Autodesk Inventor part; units mm, degrees
(part 3 of 4)
sketch "Sketch3" plane through (0, 0, 15) normal (0, 0, 1) x (1, 0, 0)
  line L0 (0, 0) -> (0, 2.4)
  line L1 (0, 2.4) -> (-384, 2.4)
  line L2 (-384, 2.4) -> (-384, 0)
  arc A0 (-384, 0) -> (-383.1122, 0.9525) centre (-384, 0.89) ccw
  arc A1 (-382.8628, 1.22) -> (-383.1122, 0.9525) centre (-382.8628, 0.97) ccw
  line L3 (-382.8628, 1.22) -> (-382.1372, 1.22)
  arc A2 (-381.8878, 0.9525) -> (-382.1372, 1.22) centre (-382.1372, 0.97) ccw
  arc A3 (-381.8878, 0.9525) -> (-380.1122, 0.9525) centre (-381, 0.89) ccw
  arc A4 (-379.8628, 1.22) -> (-380.1122, 0.9525) centre (-379.8628, 0.97) ccw
  line L4 (-379.8628, 1.22) -> (-379.1372, 1.22)
  arc A5 (-378.8878, 0.9525) -> (-379.1372, 1.22) centre (-379.1372, 0.97) ccw
  arc A6 (-378.8878, 0.9525) -> (-377.1122, 0.9525) centre (-378, 0.89) ccw
  arc A7 (-376.8628, 1.22) -> (-377.1122, 0.9525) centre (-376.8628, 0.97) ccw
  line L5 (-376.8628, 1.22) -> (-376.1372, 1.22)
  arc A8 (-375.8878, 0.9525) -> (-376.1372, 1.22) centre (-376.1372, 0.97) ccw
  arc A9 (-375.8878, 0.9525) -> (-374.1122, 0.9525) centre (-375, 0.89) ccw
  arc A10 (-373.8628, 1.22) -> (-374.1122, 0.9525) centre (-373.8628, 0.97) ccw
  line L6 (-373.8628, 1.22) -> (-373.1372, 1.22)
  arc A11 (-372.8878, 0.9525) -> (-373.1372, 1.22) centre (-373.1372, 0.97) ccw
  arc A12 (-372.8878, 0.9525) -> (-371.1122, 0.9525) centre (-372, 0.89) ccw
  arc A13 (-370.8628, 1.22) -> (-371.1122, 0.9525) centre (-370.8628, 0.97) ccw
  line L7 (-370.8628, 1.22) -> (-370.1372, 1.22)
  arc A14 (-369.8878, 0.9525) -> (-370.1372, 1.22) centre (-370.1372, 0.97) ccw
  arc A15 (-369.8878, 0.9525) -> (-368.1122, 0.9525) centre (-369, 0.89) ccw
  arc A16 (-367.8628, 1.22) -> (-368.1122, 0.9525) centre (-367.8628, 0.97) ccw
  line L8 (-367.8628, 1.22) -> (-367.1372, 1.22)
  arc A17 (-366.8878, 0.9525) -> (-367.1372, 1.22) centre (-367.1372, 0.97) ccw
  arc A18 (-366.8878, 0.9525) -> (-365.1122, 0.9525) centre (-366, 0.89) ccw
  arc A19 (-364.8628, 1.22) -> (-365.1122, 0.9525) centre (-364.8628, 0.97) ccw
  line L9 (-364.8628, 1.22) -> (-364.1372, 1.22)
  arc A20 (-363.8878, 0.9525) -> (-364.1372, 1.22) centre (-364.1372, 0.97) ccw
  arc A21 (-363.8878, 0.9525) -> (-362.1122, 0.9525) centre (-363, 0.89) ccw
  arc A22 (-361.8628, 1.22) -> (-362.1122, 0.9525) centre (-361.8628, 0.97) ccw
  line L10 (-361.8628, 1.22) -> (-361.1372, 1.22)
  arc A23 (-360.8878, 0.9525) -> (-361.1372, 1.22) centre (-361.1372, 0.97) ccw
  arc A24 (-360.8878, 0.9525) -> (-359.1122, 0.9525) centre (-360, 0.89) ccw
  arc A25 (-358.8628, 1.22) -> (-359.1122, 0.9525) centre (-358.8628, 0.97) ccw
  line L11 (-358.8628, 1.22) -> (-358.1372, 1.22)
  arc A26 (-357.8878, 0.9525) -> (-358.1372, 1.22) centre (-358.1372, 0.97) ccw
  arc A27 (-357.8878, 0.9525) -> (-356.1122, 0.9525) centre (-357, 0.89) ccw
  arc A28 (-355.8628, 1.22) -> (-356.1122, 0.9525) centre (-355.8628, 0.97) ccw
  line L12 (-355.8628, 1.22) -> (-355.1372, 1.22)
  arc A29 (-354.8878, 0.9525) -> (-355.1372, 1.22) centre (-355.1372, 0.97) ccw
  arc A30 (-354.8878, 0.9525) -> (-353.1122, 0.9525) centre (-354, 0.89) ccw
  arc A31 (-352.8628, 1.22) -> (-353.1122, 0.9525) centre (-352.8628, 0.97) ccw
  line L13 (-352.8628, 1.22) -> (-352.1372, 1.22)
  arc A32 (-351.8878, 0.9525) -> (-352.1372, 1.22) centre (-352.1372, 0.97) ccw
  arc A33 (-351.8878, 0.9525) -> (-350.1122, 0.9525) centre (-351, 0.89) ccw
  arc A34 (-349.8628, 1.22) -> (-350.1122, 0.9525) centre (-349.8628, 0.97) ccw
  line L14 (-349.8628, 1.22) -> (-349.1372, 1.22)
  arc A35 (-348.8878, 0.9525) -> (-349.1372, 1.22) centre (-349.1372, 0.97) ccw
  arc A36 (-348.8878, 0.9525) -> (-347.1122, 0.9525) centre (-348, 0.89) ccw
  arc A37 (-346.8628, 1.22) -> (-347.1122, 0.9525) centre (-346.8628, 0.97) ccw
  line L15 (-346.8628, 1.22) -> (-346.1372, 1.22)
  arc A38 (-345.8878, 0.9525) -> (-346.1372, 1.22) centre (-346.1372, 0.97) ccw
  arc A39 (-345.8878, 0.9525) -> (-344.1122, 0.9525) centre (-345, 0.89) ccw
  arc A40 (-343.8628, 1.22) -> (-344.1122, 0.9525) centre (-343.8628, 0.97) ccw
  line L16 (-343.8628, 1.22) -> (-343.1372, 1.22)
  arc A41 (-342.8878, 0.9525) -> (-343.1372, 1.22) centre (-343.1372, 0.97) ccw
  arc A42 (-342.8878, 0.9525) -> (-341.1122, 0.9525) centre (-342, 0.89) ccw
  arc A43 (-340.8628, 1.22) -> (-341.1122, 0.9525) centre (-340.8628, 0.97) ccw
  line L17 (-340.8628, 1.22) -> (-340.1372, 1.22)
  arc A44 (-339.8878, 0.9525) -> (-340.1372, 1.22) centre (-340.1372, 0.97) ccw
  arc A45 (-339.8878, 0.9525) -> (-338.1122, 0.9525) centre (-339, 0.89) ccw
  arc A46 (-337.8628, 1.22) -> (-338.1122, 0.9525) centre (-337.8628, 0.97) ccw
  line L18 (-337.8628, 1.22) -> (-337.1372, 1.22)
  arc A47 (-336.8878, 0.9525) -> (-337.1372, 1.22) centre (-337.1372, 0.97) ccw
  arc A48 (-336.8878, 0.9525) -> (-335.1122, 0.9525) centre (-336, 0.89) ccw
  arc A49 (-334.8628, 1.22) -> (-335.1122, 0.9525) centre (-334.8628, 0.97) ccw
  line L19 (-334.8628, 1.22) -> (-334.1372, 1.22)
  arc A50 (-333.8878, 0.9525) -> (-334.1372, 1.22) centre (-334.1372, 0.97) ccw
  arc A51 (-333.8878, 0.9525) -> (-332.1122, 0.9525) centre (-333, 0.89) ccw
  arc A52 (-331.8628, 1.22) -> (-332.1122, 0.9525) centre (-331.8628, 0.97) ccw
  line L20 (-331.8628, 1.22) -> (-331.1372, 1.22)
  arc A53 (-330.8878, 0.9525) -> (-331.1372, 1.22) centre (-331.1372, 0.97) ccw
  arc A54 (-330.8878, 0.9525) -> (-329.1122, 0.9525) centre (-330, 0.89) ccw
  arc A55 (-328.8628, 1.22) -> (-329.1122, 0.9525) centre (-328.8628, 0.97) ccw
  line L21 (-328.8628, 1.22) -> (-328.1372, 1.22)
  arc A56 (-327.8878, 0.9525) -> (-328.1372, 1.22) centre (-328.1372, 0.97) ccw
  arc A57 (-327.8878, 0.9525) -> (-326.1122, 0.9525) centre (-327, 0.89) ccw
  arc A58 (-325.8628, 1.22) -> (-326.1122, 0.9525) centre (-325.8628, 0.97) ccw
  line L22 (-325.8628, 1.22) -> (-325.1372, 1.22)
  arc A59 (-324.8878, 0.9525) -> (-325.1372, 1.22) centre (-325.1372, 0.97) ccw
  arc A60 (-324.8878, 0.9525) -> (-323.1122, 0.9525) centre (-324, 0.89) ccw
  arc A61 (-322.8628, 1.22) -> (-323.1122, 0.9525) centre (-322.8628, 0.97) ccw
  line L23 (-322.8628, 1.22) -> (-322.1372, 1.22)
  arc A62 (-321.8878, 0.9525) -> (-322.1372, 1.22) centre (-322.1372, 0.97) ccw
  arc A63 (-321.8878, 0.9525) -> (-320.1122, 0.9525) centre (-321, 0.89) ccw
  arc A64 (-319.8628, 1.22) -> (-320.1122, 0.9525) centre (-319.8628, 0.97) ccw
  line L24 (-319.8628, 1.22) -> (-319.1372, 1.22)
  arc A65 (-318.8878, 0.9525) -> (-319.1372, 1.22) centre (-319.1372, 0.97) ccw
  arc A66 (-318.8878, 0.9525) -> (-317.1122, 0.9525) centre (-318, 0.89) ccw
  arc A67 (-316.8628, 1.22) -> (-317.1122, 0.9525) centre (-316.8628, 0.97) ccw
  line L25 (-316.8628, 1.22) -> (-316.1372, 1.22)
  arc A68 (-315.8878, 0.9525) -> (-316.1372, 1.22) centre (-316.1372, 0.97) ccw
  arc A69 (-315.8878, 0.9525) -> (-314.1122, 0.9525) centre (-315, 0.89) ccw
  arc A70 (-313.8628, 1.22) -> (-314.1122, 0.9525) centre (-313.8628, 0.97) ccw
  line L26 (-313.8628, 1.22) -> (-313.1372, 1.22)
  arc A71 (-312.8878, 0.9525) -> (-313.1372, 1.22) centre (-313.1372, 0.97) ccw
  arc A72 (-312.8878, 0.9525) -> (-311.1122, 0.9525) centre (-312, 0.89) ccw
  arc A73 (-310.8628, 1.22) -> (-311.1122, 0.9525) centre (-310.8628, 0.97) ccw
  line L27 (-310.8628, 1.22) -> (-310.1372, 1.22)
  arc A74 (-309.8878, 0.9525) -> (-310.1372, 1.22) centre (-310.1372, 0.97) ccw
  arc A75 (-309.8878, 0.9525) -> (-308.1122, 0.9525) centre (-309, 0.89) ccw
  arc A76 (-307.8628, 1.22) -> (-308.1122, 0.9525) centre (-307.8628, 0.97) ccw
  line L28 (-307.8628, 1.22) -> (-307.1372, 1.22)
  arc A77 (-306.8878, 0.9525) -> (-307.1372, 1.22) centre (-307.1372, 0.97) ccw
  arc A78 (-306.8878, 0.9525) -> (-305.1122, 0.9525) centre (-306, 0.89) ccw
  arc A79 (-304.8628, 1.22) -> (-305.1122, 0.9525) centre (-304.8628, 0.97) ccw
  line L29 (-304.8628, 1.22) -> (-304.1372, 1.22)
  arc A80 (-303.8878, 0.9525) -> (-304.1372, 1.22) centre (-304.1372, 0.97) ccw
  arc A81 (-303.8878, 0.9525) -> (-302.1122, 0.9525) centre (-303, 0.89) ccw
  arc A82 (-301.8628, 1.22) -> (-302.1122, 0.9525) centre (-301.8628, 0.97) ccw
  line L30 (-301.8628, 1.22) -> (-301.1372, 1.22)
  arc A83 (-300.8878, 0.9525) -> (-301.1372, 1.22) centre (-301.1372, 0.97) ccw
  arc A84 (-300.8878, 0.9525) -> (-299.1122, 0.9525) centre (-300, 0.89) ccw
  arc A85 (-298.8628, 1.22) -> (-299.1122, 0.9525) centre (-298.8628, 0.97) ccw
  line L31 (-298.8628, 1.22) -> (-298.1372, 1.22)
  arc A86 (-297.8878, 0.9525) -> (-298.1372, 1.22) centre (-298.1372, 0.97) ccw
  arc A87 (-297.8878, 0.9525) -> (-296.1122, 0.9525) centre (-297, 0.89) ccw
  arc A88 (-295.8628, 1.22) -> (-296.1122, 0.9525) centre (-295.8628, 0.97) ccw
  line L32 (-295.8628, 1.22) -> (-295.1372, 1.22)
  arc A89 (-294.8878, 0.9525) -> (-295.1372, 1.22) centre (-295.1372, 0.97) ccw
  arc A90 (-294.8878, 0.9525) -> (-293.1122, 0.9525) centre (-294, 0.89) ccw
  arc A91 (-292.8628, 1.22) -> (-293.1122, 0.9525) centre (-292.8628, 0.97) ccw
  line L33 (-292.8628, 1.22) -> (-292.1372, 1.22)
  arc A92 (-291.8878, 0.9525) -> (-292.1372, 1.22) centre (-292.1372, 0.97) ccw
  arc A93 (-291.8878, 0.9525) -> (-290.1122, 0.9525) centre (-291, 0.89) ccw
  arc A94 (-289.8628, 1.22) -> (-290.1122, 0.9525) centre (-289.8628, 0.97) ccw
  line L34 (-289.8628, 1.22) -> (-289.1372, 1.22)
  arc A95 (-288.8878, 0.9525) -> (-289.1372, 1.22) centre (-289.1372, 0.97) ccw
  arc A96 (-288.8878, 0.9525) -> (-287.1122, 0.9525) centre (-288, 0.89) ccw
  arc A97 (-286.8628, 1.22) -> (-287.1122, 0.9525) centre (-286.8628, 0.97) ccw
  line L35 (-286.8628, 1.22) -> (-286.1372, 1.22)
  arc A98 (-285.8878, 0.9525) -> (-286.1372, 1.22) centre (-286.1372, 0.97) ccw
  arc A99 (-285.8878, 0.9525) -> (-284.1122, 0.9525) centre (-285, 0.89) ccw
  arc A100 (-283.8628, 1.22) -> (-284.1122, 0.9525) centre (-283.8628, 0.97) ccw
  line L36 (-283.8628, 1.22) -> (-283.1372, 1.22)
  arc A101 (-282.8878, 0.9525) -> (-283.1372, 1.22) centre (-283.1372, 0.97) ccw
  arc A102 (-282.8878, 0.9525) -> (-281.1122, 0.9525) centre (-282, 0.89) ccw
  arc A103 (-280.8628, 1.22) -> (-281.1122, 0.9525) centre (-280.8628, 0.97) ccw
  line L37 (-280.8628, 1.22) -> (-280.1372, 1.22)
  arc A104 (-279.8878, 0.9525) -> (-280.1372, 1.22) centre (-280.1372, 0.97) ccw
  arc A105 (-279.8878, 0.9525) -> (-278.1122, 0.9525) centre (-279, 0.89) ccw
  arc A106 (-277.8628, 1.22) -> (-278.1122, 0.9525) centre (-277.8628, 0.97) ccw
  line L38 (-277.8628, 1.22) -> (-277.1372, 1.22)
  arc A107 (-276.8878, 0.9525) -> (-277.1372, 1.22) centre (-277.1372, 0.97) ccw
  arc A108 (-276.8878, 0.9525) -> (-275.1122, 0.9525) centre (-276, 0.89) ccw
  arc A109 (-274.8628, 1.22) -> (-275.1122, 0.9525) centre (-274.8628, 0.97) ccw
  line L39 (-274.8628, 1.22) -> (-274.1372, 1.22)
  arc A110 (-273.8878, 0.9525) -> (-274.1372, 1.22) centre (-274.1372, 0.97) ccw
  arc A111 (-273.8878, 0.9525) -> (-272.1122, 0.9525) centre (-273, 0.89) ccw
  arc A112 (-271.8628, 1.22) -> (-272.1122, 0.9525) centre (-271.8628, 0.97) ccw
  line L40 (-271.8628, 1.22) -> (-271.1372, 1.22)
  arc A113 (-270.8878, 0.9525) -> (-271.1372, 1.22) centre (-271.1372, 0.97) ccw
  arc A114 (-270.8878, 0.9525) -> (-269.1122, 0.9525) centre (-270, 0.89) ccw
  arc A115 (-268.8628, 1.22) -> (-269.1122, 0.9525) centre (-268.8628, 0.97) ccw
  line L41 (-268.8628, 1.22) -> (-268.1372, 1.22)
  arc A116 (-267.8878, 0.9525) -> (-268.1372, 1.22) centre (-268.1372, 0.97) ccw
  arc A117 (-267.8878, 0.9525) -> (-266.1122, 0.9525) centre (-267, 0.89) ccw
  arc A118 (-265.8628, 1.22) -> (-266.1122, 0.9525) centre (-265.8628, 0.97) ccw
  line L42 (-265.8628, 1.22) -> (-265.1372, 1.22)
  arc A119 (-264.8878, 0.9525) -> (-265.1372, 1.22) centre (-265.1372, 0.97) ccw
  arc A120 (-264.8878, 0.9525) -> (-263.1122, 0.9525) centre (-264, 0.89) ccw
  arc A121 (-262.8628, 1.22) -> (-263.1122, 0.9525) centre (-262.8628, 0.97) ccw
  line L43 (-262.8628, 1.22) -> (-262.1372, 1.22)
  arc A122 (-261.8878, 0.9525) -> (-262.1372, 1.22) centre (-262.1372, 0.97) ccw
  arc A123 (-261.8878, 0.9525) -> (-260.1122, 0.9525) centre (-261, 0.89) ccw
  arc A124 (-259.8628, 1.22) -> (-260.1122, 0.9525) centre (-259.8628, 0.97) ccw
  line L44 (-259.8628, 1.22) -> (-259.1372, 1.22)
  arc A125 (-258.8878, 0.9525) -> (-259.1372, 1.22) centre (-259.1372, 0.97) ccw
  arc A126 (-258.8878, 0.9525) -> (-257.1122, 0.9525) centre (-258, 0.89) ccw
  arc A127 (-256.8628, 1.22) -> (-257.1122, 0.9525) centre (-256.8628, 0.97) ccw
  line L45 (-256.8628, 1.22) -> (-256.1372, 1.22)
  arc A128 (-255.8878, 0.9525) -> (-256.1372, 1.22) centre (-256.1372, 0.97) ccw
  arc A129 (-255.8878, 0.9525) -> (-254.1122, 0.9525) centre (-255, 0.89) ccw
  arc A130 (-253.8628, 1.22) -> (-254.1122, 0.9525) centre (-253.8628, 0.97) ccw
  line L46 (-253.8628, 1.22) -> (-253.1372, 1.22)
  arc A131 (-252.8878, 0.9525) -> (-253.1372, 1.22) centre (-253.1372, 0.97) ccw
  arc A132 (-252.8878, 0.9525) -> (-251.1122, 0.9525) centre (-252, 0.89) ccw
  arc A133 (-250.8628, 1.22) -> (-251.1122, 0.9525) centre (-250.8628, 0.97) ccw
  line L47 (-250.8628, 1.22) -> (-250.1372, 1.22)
  arc A134 (-249.8878, 0.9525) -> (-250.1372, 1.22) centre (-250.1372, 0.97) ccw
  arc A135 (-249.8878, 0.9525) -> (-248.1122, 0.9525) centre (-249, 0.89) ccw
  arc A136 (-247.8628, 1.22) -> (-248.1122, 0.9525) centre (-247.8628, 0.97) ccw
  line L48 (-247.8628, 1.22) -> (-247.1372, 1.22)
  arc A137 (-246.8878, 0.9525) -> (-247.1372, 1.22) centre (-247.1372, 0.97) ccw
  arc A138 (-246.8878, 0.9525) -> (-245.1122, 0.9525) centre (-246, 0.89) ccw
  arc A139 (-244.8628, 1.22) -> (-245.1122, 0.9525) centre (-244.8628, 0.97) ccw
  line L49 (-244.8628, 1.22) -> (-244.1372, 1.22)
  arc A140 (-243.8878, 0.9525) -> (-244.1372, 1.22) centre (-244.1372, 0.97) ccw
  arc A141 (-243.8878, 0.9525) -> (-242.1122, 0.9525) centre (-243, 0.89) ccw
  arc A142 (-241.8628, 1.22) -> (-242.1122, 0.9525) centre (-241.8628, 0.97) ccw
  line L50 (-241.8628, 1.22) -> (-241.1372, 1.22)
  arc A143 (-240.8878, 0.9525) -> (-241.1372, 1.22) centre (-241.1372, 0.97) ccw
  arc A144 (-240.8878, 0.9525) -> (-239.1122, 0.9525) centre (-240, 0.89) ccw
  arc A145 (-238.8628, 1.22) -> (-239.1122, 0.9525) centre (-238.8628, 0.97) ccw
  line L51 (-238.8628, 1.22) -> (-238.1372, 1.22)
  arc A146 (-237.8878, 0.9525) -> (-238.1372, 1.22) centre (-238.1372, 0.97) ccw
  arc A147 (-237.8878, 0.9525) -> (-236.1122, 0.9525) centre (-237, 0.89) ccw
  arc A148 (-235.8628, 1.22) -> (-236.1122, 0.9525) centre (-235.8628, 0.97) ccw
  line L52 (-235.8628, 1.22) -> (-235.1372, 1.22)
  arc A149 (-234.8878, 0.9525) -> (-235.1372, 1.22) centre (-235.1372, 0.97) ccw
  arc A150 (-234.8878, 0.9525) -> (-233.1122, 0.9525) centre (-234, 0.89) ccw
  arc A151 (-232.8628, 1.22) -> (-233.1122, 0.9525) centre (-232.8628, 0.97) ccw
  line L53 (-232.8628, 1.22) -> (-232.1372, 1.22)
  arc A152 (-231.8878, 0.9525) -> (-232.1372, 1.22) centre (-232.1372, 0.97) ccw
  arc A153 (-231.8878, 0.9525) -> (-230.1122, 0.9525) centre (-231, 0.89) ccw
  arc A154 (-229.8628, 1.22) -> (-230.1122, 0.9525) centre (-229.8628, 0.97) ccw
  line L54 (-229.8628, 1.22) -> (-229.1372, 1.22)
  arc A155 (-228.8878, 0.9525) -> (-229.1372, 1.22) centre (-229.1372, 0.97) ccw
  arc A156 (-228.8878, 0.9525) -> (-227.1122, 0.9525) centre (-228, 0.89) ccw
  arc A157 (-226.8628, 1.22) -> (-227.1122, 0.9525) centre (-226.8628, 0.97) ccw
  line L55 (-226.8628, 1.22) -> (-226.1372, 1.22)
  arc A158 (-225.8878, 0.9525) -> (-226.1372, 1.22) centre (-226.1372, 0.97) ccw
  arc A159 (-225.8878, 0.9525) -> (-224.1122, 0.9525) centre (-225, 0.89) ccw
  arc A160 (-223.8628, 1.22) -> (-224.1122, 0.9525) centre (-223.8628, 0.97) ccw
  line L56 (-223.8628, 1.22) -> (-223.1372, 1.22)
  arc A161 (-222.8878, 0.9525) -> (-223.1372, 1.22) centre (-223.1372, 0.97) ccw
  arc A162 (-222.8878, 0.9525) -> (-221.1122, 0.9525) centre (-222, 0.89) ccw
  arc A163 (-220.8628, 1.22) -> (-221.1122, 0.9525) centre (-220.8628, 0.97) ccw
  line L57 (-220.8628, 1.22) -> (-220.1372, 1.22)
  arc A164 (-219.8878, 0.9525) -> (-220.1372, 1.22) centre (-220.1372, 0.97) ccw
  arc A165 (-219.8878, 0.9525) -> (-218.1122, 0.9525) centre (-219, 0.89) ccw
  arc A166 (-217.8628, 1.22) -> (-218.1122, 0.9525) centre (-217.8628, 0.97) ccw
  line L58 (-217.8628, 1.22) -> (-217.1372, 1.22)
  arc A167 (-216.8878, 0.9525) -> (-217.1372, 1.22) centre (-217.1372, 0.97) ccw
  arc A168 (-216.8878, 0.9525) -> (-215.1122, 0.9525) centre (-216, 0.89) ccw
  arc A169 (-214.8628, 1.22) -> (-215.1122, 0.9525) centre (-214.8628, 0.97) ccw
  line L59 (-214.8628, 1.22) -> (-214.1372, 1.22)
  arc A170 (-213.8878, 0.9525) -> (-214.1372, 1.22) centre (-214.1372, 0.97) ccw
  arc A171 (-213.8878, 0.9525) -> (-212.1122, 0.9525) centre (-213, 0.89) ccw
  arc A172 (-211.8628, 1.22) -> (-212.1122, 0.9525) centre (-211.8628, 0.97) ccw
  line L60 (-211.8628, 1.22) -> (-211.1372, 1.22)
  arc A173 (-210.8878, 0.9525) -> (-211.1372, 1.22) centre (-211.1372, 0.97) ccw
  arc A174 (-210.8878, 0.9525) -> (-209.1122, 0.9525) centre (-210, 0.89) ccw
  arc A175 (-208.8628, 1.22) -> (-209.1122, 0.9525) centre (-208.8628, 0.97) ccw
  line L61 (-208.8628, 1.22) -> (-208.1372, 1.22)
  arc A176 (-207.8878, 0.9525) -> (-208.1372, 1.22) centre (-208.1372, 0.97) ccw
  arc A177 (-207.8878, 0.9525) -> (-206.1122, 0.9525) centre (-207, 0.89) ccw
  arc A178 (-205.8628, 1.22) -> (-206.1122, 0.9525) centre (-205.8628, 0.97) ccw
  line L62 (-205.8628, 1.22) -> (-205.1372, 1.22)
  arc A179 (-204.8878, 0.9525) -> (-205.1372, 1.22) centre (-205.1372, 0.97) ccw
  arc A180 (-204.8878, 0.9525) -> (-203.1122, 0.9525) centre (-204, 0.89) ccw
  arc A181 (-202.8628, 1.22) -> (-203.1122, 0.9525) centre (-202.8628, 0.97) ccw
  line L63 (-202.8628, 1.22) -> (-202.1372, 1.22)
  arc A182 (-201.8878, 0.9525) -> (-202.1372, 1.22) centre (-202.1372, 0.97) ccw
  arc A183 (-201.8878, 0.9525) -> (-200.1122, 0.9525) centre (-201, 0.89) ccw
  arc A184 (-199.8628, 1.22) -> (-200.1122, 0.9525) centre (-199.8628, 0.97) ccw
  line L64 (-199.8628, 1.22) -> (-199.1372, 1.22)
  arc A185 (-198.8878, 0.9525) -> (-199.1372, 1.22) centre (-199.1372, 0.97) ccw
  arc A186 (-198.8878, 0.9525) -> (-197.1122, 0.9525) centre (-198, 0.89) ccw
  arc A187 (-196.8628, 1.22) -> (-197.1122, 0.9525) centre (-196.8628, 0.97) ccw
  line L65 (-196.8628, 1.22) -> (-196.1372, 1.22)
  arc A188 (-195.8878, 0.9525) -> (-196.1372, 1.22) centre (-196.1372, 0.97) ccw
  arc A189 (-195.8878, 0.9525) -> (-194.1122, 0.9525) centre (-195, 0.89) ccw
  arc A190 (-193.8628, 1.22) -> (-194.1122, 0.9525) centre (-193.8628, 0.97) ccw
  line L66 (-193.8628, 1.22) -> (-193.1372, 1.22)
  arc A191 (-192.8878, 0.9525) -> (-193.1372, 1.22) centre (-193.1372, 0.97) ccw
  arc A192 (-192.8878, 0.9525) -> (-191.1122, 0.9525) centre (-192, 0.89) ccw
  arc A193 (-190.8628, 1.22) -> (-191.1122, 0.9525) centre (-190.8628, 0.97) ccw
  line L67 (-190.8628, 1.22) -> (-190.1372, 1.22)
  arc A194 (-189.8878, 0.9525) -> (-190.1372, 1.22) centre (-190.1372, 0.97) ccw
  arc A195 (-189.8878, 0.9525) -> (-188.1122, 0.9525) centre (-189, 0.89) ccw
  arc A196 (-187.8628, 1.22) -> (-188.1122, 0.9525) centre (-187.8628, 0.97) ccw
  line L68 (-187.8628, 1.22) -> (-187.1372, 1.22)
  arc A197 (-186.8878, 0.9525) -> (-187.1372, 1.22) centre (-187.1372, 0.97) ccw
  arc A198 (-186.8878, 0.9525) -> (-185.1122, 0.9525) centre (-186, 0.89) ccw
  arc A199 (-184.8628, 1.22) -> (-185.1122, 0.9525) centre (-184.8628, 0.97) ccw
  line L69 (-184.8628, 1.22) -> (-184.1372, 1.22)
  arc A200 (-183.8878, 0.9525) -> (-184.1372, 1.22) centre (-184.1372, 0.97) ccw
  arc A201 (-183.8878, 0.9525) -> (-182.1122, 0.9525) centre (-183, 0.89) ccw
  arc A202 (-181.8628, 1.22) -> (-182.1122, 0.9525) centre (-181.8628, 0.97) ccw
  line L70 (-181.8628, 1.22) -> (-181.1372, 1.22)
  arc A203 (-180.8878, 0.9525) -> (-181.1372, 1.22) centre (-181.1372, 0.97) ccw
  arc A204 (-180.8878, 0.9525) -> (-179.1122, 0.9525) centre (-180, 0.89) ccw
  arc A205 (-178.8628, 1.22) -> (-179.1122, 0.9525) centre (-178.8628, 0.97) ccw
  line L71 (-178.8628, 1.22) -> (-178.1372, 1.22)
  arc A206 (-177.8878, 0.9525) -> (-178.1372, 1.22) centre (-178.1372, 0.97) ccw
  arc A207 (-177.8878, 0.9525) -> (-176.1122, 0.9525) centre (-177, 0.89) ccw
  arc A208 (-175.8628, 1.22) -> (-176.1122, 0.9525) centre (-175.8628, 0.97) ccw
  line L72 (-175.8628, 1.22) -> (-175.1372, 1.22)
  arc A209 (-174.8878, 0.9525) -> (-175.1372, 1.22) centre (-175.1372, 0.97) ccw
  arc A210 (-174.8878, 0.9525) -> (-173.1122, 0.9525) centre (-174, 0.89) ccw
  arc A211 (-172.8628, 1.22) -> (-173.1122, 0.9525) centre (-172.8628, 0.97) ccw
  line L73 (-172.8628, 1.22) -> (-172.1372, 1.22)
  arc A212 (-171.8878, 0.9525) -> (-172.1372, 1.22) centre (-172.1372, 0.97) ccw
  arc A213 (-171.8878, 0.9525) -> (-170.1122, 0.9525) centre (-171, 0.89) ccw
  arc A214 (-169.8628, 1.22) -> (-170.1122, 0.9525) centre (-169.8628, 0.97) ccw
  line L74 (-169.8628, 1.22) -> (-169.1372, 1.22)
  arc A215 (-168.8878, 0.9525) -> (-169.1372, 1.22) centre (-169.1372, 0.97) ccw
  arc A216 (-168.8878, 0.9525) -> (-167.1122, 0.9525) centre (-168, 0.89) ccw
  arc A217 (-166.8628, 1.22) -> (-167.1122, 0.9525) centre (-166.8628, 0.97) ccw
  line L75 (-166.8628, 1.22) -> (-166.1372, 1.22)
  arc A218 (-165.8878, 0.9525) -> (-166.1372, 1.22) centre (-166.1372, 0.97) ccw
  arc A219 (-165.8878, 0.9525) -> (-164.1122, 0.9525) centre (-165, 0.89) ccw
  arc A220 (-163.8628, 1.22) -> (-164.1122, 0.9525) centre (-163.8628, 0.97) ccw
  line L76 (-163.8628, 1.22) -> (-163.1372, 1.22)
  arc A221 (-162.8878, 0.9525) -> (-163.1372, 1.22) centre (-163.1372, 0.97) ccw
  arc A222 (-162.8878, 0.9525) -> (-161.1122, 0.9525) centre (-162, 0.89) ccw
  arc A223 (-160.8628, 1.22) -> (-161.1122, 0.9525) centre (-160.8628, 0.97) ccw
  line L77 (-160.8628, 1.22) -> (-160.1372, 1.22)
  arc A224 (-159.8878, 0.9525) -> (-160.1372, 1.22) centre (-160.1372, 0.97) ccw
  arc A225 (-159.8878, 0.9525) -> (-158.1122, 0.9525) centre (-159, 0.89) ccw
  arc A226 (-157.8628, 1.22) -> (-158.1122, 0.9525) centre (-157.8628, 0.97) ccw
  line L78 (-157.8628, 1.22) -> (-157.1372, 1.22)
  arc A227 (-156.8878, 0.9525) -> (-157.1372, 1.22) centre (-157.1372, 0.97) ccw
  arc A228 (-156.8878, 0.9525) -> (-155.1122, 0.9525) centre (-156, 0.89) ccw
  arc A229 (-154.8628, 1.22) -> (-155.1122, 0.9525) centre (-154.8628, 0.97) ccw
  line L79 (-154.8628, 1.22) -> (-154.1372, 1.22)
  arc A230 (-153.8878, 0.9525) -> (-154.1372, 1.22) centre (-154.1372, 0.97) ccw
  arc A231 (-153.8878, 0.9525) -> (-152.1122, 0.9525) centre (-153, 0.89) ccw
  arc A232 (-151.8628, 1.22) -> (-152.1122, 0.9525) centre (-151.8628, 0.97) ccw
  line L80 (-151.8628, 1.22) -> (-151.1372, 1.22)
  arc A233 (-150.8878, 0.9525) -> (-151.1372, 1.22) centre (-151.1372, 0.97) ccw
  arc A234 (-150.8878, 0.9525) -> (-149.1122, 0.9525) centre (-150, 0.89) ccw
  arc A235 (-148.8628, 1.22) -> (-149.1122, 0.9525) centre (-148.8628, 0.97) ccw
  line L81 (-148.8628, 1.22) -> (-148.1372, 1.22)
  arc A236 (-147.8878, 0.9525) -> (-148.1372, 1.22) centre (-148.1372, 0.97) ccw
  arc A237 (-147.8878, 0.9525) -> (-146.1122, 0.9525) centre (-147, 0.89) ccw
  arc A238 (-145.8628, 1.22) -> (-146.1122, 0.9525) centre (-145.8628, 0.97) ccw
  line L82 (-145.8628, 1.22) -> (-145.1372, 1.22)
  arc A239 (-144.8878, 0.9525) -> (-145.1372, 1.22) centre (-145.1372, 0.97) ccw
  arc A240 (-144.8878, 0.9525) -> (-143.1122, 0.9525) centre (-144, 0.89) ccw
  arc A241 (-142.8628, 1.22) -> (-143.1122, 0.9525) centre (-142.8628, 0.97) ccw
  line L83 (-142.8628, 1.22) -> (-142.1372, 1.22)
  arc A242 (-141.8878, 0.9525) -> (-142.1372, 1.22) centre (-142.1372, 0.97) ccw
  arc A243 (-141.8878, 0.9525) -> (-140.1122, 0.9525) centre (-141, 0.89) ccw
  arc A244 (-139.8628, 1.22) -> (-140.1122, 0.9525) centre (-139.8628, 0.97) ccw
  line L84 (-139.8628, 1.22) -> (-139.1372, 1.22)
  arc A245 (-138.8878, 0.9525) -> (-139.1372, 1.22) centre (-139.1372, 0.97) ccw
  arc A246 (-138.8878, 0.9525) -> (-137.1122, 0.9525) centre (-138, 0.89) ccw
  arc A247 (-136.8628, 1.22) -> (-137.1122, 0.9525) centre (-136.8628, 0.97) ccw
  line L85 (-136.8628, 1.22) -> (-136.1372, 1.22)
  arc A248 (-135.8878, 0.9525) -> (-136.1372, 1.22) centre (-136.1372, 0.97) ccw
  arc A249 (-135.8878, 0.9525) -> (-134.1122, 0.9525) centre (-135, 0.89) ccw
  arc A250 (-133.8628, 1.22) -> (-134.1122, 0.9525) centre (-133.8628, 0.97) ccw
  line L86 (-133.8628, 1.22) -> (-133.1372, 1.22)
  arc A251 (-132.8878, 0.9525) -> (-133.1372, 1.22) centre (-133.1372, 0.97) ccw
  arc A252 (-132.8878, 0.9525) -> (-131.1122, 0.9525) centre (-132, 0.89) ccw
  arc A253 (-130.8628, 1.22) -> (-131.1122, 0.9525) centre (-130.8628, 0.97) ccw
  line L87 (-130.8628, 1.22) -> (-130.1372, 1.22)
  arc A254 (-129.8878, 0.9525) -> (-130.1372, 1.22) centre (-130.1372, 0.97) ccw
  arc A255 (-129.8878, 0.9525) -> (-128.1122, 0.9525) centre (-129, 0.89) ccw
  arc A256 (-127.8628, 1.22) -> (-128.1122, 0.9525) centre (-127.8628, 0.97) ccw
  line L88 (-127.8628, 1.22) -> (-127.1372, 1.22)
  arc A257 (-126.8878, 0.9525) -> (-127.1372, 1.22) centre (-127.1372, 0.97) ccw
  arc A258 (-126.8878, 0.9525) -> (-125.1122, 0.9525) centre (-126, 0.89) ccw
  arc A259 (-124.8628, 1.22) -> (-125.1122, 0.9525) centre (-124.8628, 0.97) ccw
  line L89 (-124.8628, 1.22) -> (-124.1372, 1.22)
  arc A260 (-123.8878, 0.9525) -> (-124.1372, 1.22) centre (-124.1372, 0.97) ccw
  arc A261 (-123.8878, 0.9525) -> (-122.1122, 0.9525) centre (-123, 0.89) ccw
  arc A262 (-121.8628, 1.22) -> (-122.1122, 0.9525) centre (-121.8628, 0.97) ccw
  line L90 (-121.8628, 1.22) -> (-121.1372, 1.22)
  arc A263 (-120.8878, 0.9525) -> (-121.1372, 1.22) centre (-121.1372, 0.97) ccw
  arc A264 (-120.8878, 0.9525) -> (-119.1122, 0.9525) centre (-120, 0.89) ccw
  arc A265 (-118.8628, 1.22) -> (-119.1122, 0.9525) centre (-118.8628, 0.97) ccw
  line L91 (-118.8628, 1.22) -> (-118.1372, 1.22)
  arc A266 (-117.8878, 0.9525) -> (-118.1372, 1.22) centre (-118.1372, 0.97) ccw
  arc A267 (-117.8878, 0.9525) -> (-116.1122, 0.9525) centre (-117, 0.89) ccw
  arc A268 (-115.8628, 1.22) -> (-116.1122, 0.9525) centre (-115.8628, 0.97) ccw
  line L92 (-115.8628, 1.22) -> (-115.1372, 1.22)
  arc A269 (-114.8878, 0.9525) -> (-115.1372, 1.22) centre (-115.1372, 0.97) ccw
  arc A270 (-114.8878, 0.9525) -> (-113.1122, 0.9525) centre (-114, 0.89) ccw
  arc A271 (-112.8628, 1.22) -> (-113.1122, 0.9525) centre (-112.8628, 0.97) ccw
  line L93 (-112.8628, 1.22) -> (-112.1372, 1.22)
  arc A272 (-111.8878, 0.9525) -> (-112.1372, 1.22) centre (-112.1372, 0.97) ccw
  arc A273 (-111.8878, 0.9525) -> (-110.1122, 0.9525) centre (-111, 0.89) ccw
  arc A274 (-109.8628, 1.22) -> (-110.1122, 0.9525) centre (-109.8628, 0.97) ccw
  line L94 (-109.8628, 1.22) -> (-109.1372, 1.22)
  arc A275 (-108.8878, 0.9525) -> (-109.1372, 1.22) centre (-109.1372, 0.97) ccw
  arc A276 (-108.8878, 0.9525) -> (-107.1122, 0.9525) centre (-108, 0.89) ccw
  arc A277 (-106.8628, 1.22) -> (-107.1122, 0.9525) centre (-106.8628, 0.97) ccw
  line L95 (-106.8628, 1.22) -> (-106.1372, 1.22)
  arc A278 (-105.8878, 0.9525) -> (-106.1372, 1.22) centre (-106.1372, 0.97) ccw
  arc A279 (-105.8878, 0.9525) -> (-104.1122, 0.9525) centre (-105, 0.89) ccw
  arc A280 (-103.8628, 1.22) -> (-104.1122, 0.9525) centre (-103.8628, 0.97) ccw
  line L96 (-103.8628, 1.22) -> (-103.1372, 1.22)
  arc A281 (-102.8878, 0.9525) -> (-103.1372, 1.22) centre (-103.1372, 0.97) ccw
  arc A282 (-102.8878, 0.9525) -> (-101.1122, 0.9525) centre (-102, 0.89) ccw
  arc A283 (-100.8628, 1.22) -> (-101.1122, 0.9525) centre (-100.8628, 0.97) ccw
  line L97 (-100.8628, 1.22) -> (-100.1372, 1.22)
  arc A284 (-99.8878, 0.9525) -> (-100.1372, 1.22) centre (-100.1372, 0.97) ccw
  arc A285 (-99.8878, 0.9525) -> (-98.1122, 0.9525) centre (-99, 0.89) ccw
  arc A286 (-97.8628, 1.22) -> (-98.1122, 0.9525) centre (-97.8628, 0.97) ccw
  line L98 (-97.8628, 1.22) -> (-97.1372, 1.22)
  arc A287 (-96.8878, 0.9525) -> (-97.1372, 1.22) centre (-97.1372, 0.97) ccw
  arc A288 (-96.8878, 0.9525) -> (-95.1122, 0.9525) centre (-96, 0.89) ccw
  arc A289 (-94.8628, 1.22) -> (-95.1122, 0.9525) centre (-94.8628, 0.97) ccw
  line L99 (-94.8628, 1.22) -> (-94.1372, 1.22)
  arc A290 (-93.8878, 0.9525) -> (-94.1372, 1.22) centre (-94.1372, 0.97) ccw
  arc A291 (-93.8878, 0.9525) -> (-92.1122, 0.9525) centre (-93, 0.89) ccw
  arc A292 (-91.8628, 1.22) -> (-92.1122, 0.9525) centre (-91.8628, 0.97) ccw
  line L100 (-91.8628, 1.22) -> (-91.1372, 1.22)
  arc A293 (-90.8878, 0.9525) -> (-91.1372, 1.22) centre (-91.1372, 0.97) ccw
  arc A294 (-90.8878, 0.9525) -> (-89.1122, 0.9525) centre (-90, 0.89) ccw
  arc A295 (-88.8628, 1.22) -> (-89.1122, 0.9525) centre (-88.8628, 0.97) ccw
  line L101 (-88.8628, 1.22) -> (-88.1372, 1.22)
  arc A296 (-87.8878, 0.9525) -> (-88.1372, 1.22) centre (-88.1372, 0.97) ccw
  arc A297 (-87.8878, 0.9525) -> (-86.1122, 0.9525) centre (-87, 0.89) ccw
  arc A298 (-85.8628, 1.22) -> (-86.1122, 0.9525) centre (-85.8628, 0.97) ccw
  line L102 (-85.8628, 1.22) -> (-85.1372, 1.22)
  arc A299 (-84.8878, 0.9525) -> (-85.1372, 1.22) centre (-85.1372, 0.97) ccw
  arc A300 (-84.8878, 0.9525) -> (-83.1122, 0.9525) centre (-84, 0.89) ccw
  arc A301 (-82.8628, 1.22) -> (-83.1122, 0.9525) centre (-82.8628, 0.97) ccw
  line L103 (-82.8628, 1.22) -> (-82.1372, 1.22)
  arc A302 (-81.8878, 0.9525) -> (-82.1372, 1.22) centre (-82.1372, 0.97) ccw
  arc A303 (-81.8878, 0.9525) -> (-80.1122, 0.9525) centre (-81, 0.89) ccw
  arc A304 (-79.8628, 1.22) -> (-80.1122, 0.9525) centre (-79.8628, 0.97) ccw
  line L104 (-79.8628, 1.22) -> (-79.1372, 1.22)
  arc A305 (-78.8878, 0.9525) -> (-79.1372, 1.22) centre (-79.1372, 0.97) ccw
  arc A306 (-78.8878, 0.9525) -> (-77.1122, 0.9525) centre (-78, 0.89) ccw
  arc A307 (-76.8628, 1.22) -> (-77.1122, 0.9525) centre (-76.8628, 0.97) ccw
  line L105 (-76.8628, 1.22) -> (-76.1372, 1.22)
  arc A308 (-75.8878, 0.9525) -> (-76.1372, 1.22) centre (-76.1372, 0.97) ccw
  arc A309 (-75.8878, 0.9525) -> (-74.1122, 0.9525) centre (-75, 0.89) ccw
  arc A310 (-73.8628, 1.22) -> (-74.1122, 0.9525) centre (-73.8628, 0.97) ccw
  line L106 (-73.8628, 1.22) -> (-73.1372, 1.22)
  arc A311 (-72.8878, 0.9525) -> (-73.1372, 1.22) centre (-73.1372, 0.97) ccw
  arc A312 (-72.8878, 0.9525) -> (-71.1122, 0.9525) centre (-72, 0.89) ccw
  arc A313 (-70.8628, 1.22) -> (-71.1122, 0.9525) centre (-70.8628, 0.97) ccw
  line L107 (-70.8628, 1.22) -> (-70.1372, 1.22)
  arc A314 (-69.8878, 0.9525) -> (-70.1372, 1.22) centre (-70.1372, 0.97) ccw
  arc A315 (-69.8878, 0.9525) -> (-68.1122, 0.9525) centre (-69, 0.89) ccw
  arc A316 (-67.8628, 1.22) -> (-68.1122, 0.9525) centre (-67.8628, 0.97) ccw
  line L108 (-67.8628, 1.22) -> (-67.1372, 1.22)
  arc A317 (-66.8878, 0.9525) -> (-67.1372, 1.22) centre (-67.1372, 0.97) ccw
  arc A318 (-66.8878, 0.9525) -> (-65.1122, 0.9525) centre (-66, 0.89) ccw
  arc A319 (-64.8628, 1.22) -> (-65.1122, 0.9525) centre (-64.8628, 0.97) ccw
  line L109 (-64.8628, 1.22) -> (-64.1372, 1.22)
  arc A320 (-63.8878, 0.9525) -> (-64.1372, 1.22) centre (-64.1372, 0.97) ccw
  arc A321 (-63.8878, 0.9525) -> (-62.1122, 0.9525) centre (-63, 0.89) ccw
  arc A322 (-61.8628, 1.22) -> (-62.1122, 0.9525) centre (-61.8628, 0.97) ccw
  line L110 (-61.8628, 1.22) -> (-61.1372, 1.22)
  arc A323 (-60.8878, 0.9525) -> (-61.1372, 1.22) centre (-61.1372, 0.97) ccw
  arc A324 (-60.8878, 0.9525) -> (-59.1122, 0.9525) centre (-60, 0.89) ccw
  arc A325 (-58.8628, 1.22) -> (-59.1122, 0.9525) centre (-58.8628, 0.97) ccw
  line L111 (-58.8628, 1.22) -> (-58.1372, 1.22)
  arc A326 (-57.8878, 0.9525) -> (-58.1372, 1.22) centre (-58.1372, 0.97) ccw
  arc A327 (-57.8878, 0.9525) -> (-56.1122, 0.9525) centre (-57, 0.89) ccw
  arc A328 (-55.8628, 1.22) -> (-56.1122, 0.9525) centre (-55.8628, 0.97) ccw
  line L112 (-55.8628, 1.22) -> (-55.1372, 1.22)
  arc A329 (-54.8878, 0.9525) -> (-55.1372, 1.22) centre (-55.1372, 0.97) ccw
  arc A330 (-54.8878, 0.9525) -> (-53.1122, 0.9525) centre (-54, 0.89) ccw
  arc A331 (-52.8628, 1.22) -> (-53.1122, 0.9525) centre (-52.8628, 0.97) ccw
  line L113 (-52.8628, 1.22) -> (-52.1372, 1.22)
  arc A332 (-51.8878, 0.9525) -> (-52.1372, 1.22) centre (-52.1372, 0.97) ccw
  arc A333 (-51.8878, 0.9525) -> (-50.1122, 0.9525) centre (-51, 0.89) ccw
  arc A334 (-49.8628, 1.22) -> (-50.1122, 0.9525) centre (-49.8628, 0.97) ccw
  line L114 (-49.8628, 1.22) -> (-49.1372, 1.22)
  arc A335 (-48.8878, 0.9525) -> (-49.1372, 1.22) centre (-49.1372, 0.97) ccw
  arc A336 (-48.8878, 0.9525) -> (-47.1122, 0.9525) centre (-48, 0.89) ccw
  arc A337 (-46.8628, 1.22) -> (-47.1122, 0.9525) centre (-46.8628, 0.97) ccw
  line L115 (-46.8628, 1.22) -> (-46.1372, 1.22)
  arc A338 (-45.8878, 0.9525) -> (-46.1372, 1.22) centre (-46.1372, 0.97) ccw
  arc A339 (-45.8878, 0.9525) -> (-44.1122, 0.9525) centre (-45, 0.89) ccw
  arc A340 (-43.8628, 1.22) -> (-44.1122, 0.9525) centre (-43.8628, 0.97) ccw
  line L116 (-43.8628, 1.22) -> (-43.1372, 1.22)
  arc A341 (-42.8878, 0.9525) -> (-43.1372, 1.22) centre (-43.1372, 0.97) ccw
  arc A342 (-42.8878, 0.9525) -> (-41.1122, 0.9525) centre (-42, 0.89) ccw
  arc A343 (-40.8628, 1.22) -> (-41.1122, 0.9525) centre (-40.8628, 0.97) ccw
  line L117 (-40.8628, 1.22) -> (-40.1372, 1.22)
  arc A344 (-39.8878, 0.9525) -> (-40.1372, 1.22) centre (-40.1372, 0.97) ccw
  arc A345 (-39.8878, 0.9525) -> (-38.1122, 0.9525) centre (-39, 0.89) ccw
  arc A346 (-37.8628, 1.22) -> (-38.1122, 0.9525) centre (-37.8628, 0.97) ccw
  line L118 (-37.8628, 1.22) -> (-37.1372, 1.22)
  arc A347 (-36.8878, 0.9525) -> (-37.1372, 1.22) centre (-37.1372, 0.97) ccw
  arc A348 (-36.8878, 0.9525) -> (-35.1122, 0.9525) centre (-36, 0.89) ccw
  arc A349 (-34.8628, 1.22) -> (-35.1122, 0.9525) centre (-34.8628, 0.97) ccw
  line L119 (-34.8628, 1.22) -> (-34.1372, 1.22)
  arc A350 (-33.8878, 0.9525) -> (-34.1372, 1.22) centre (-34.1372, 0.97) ccw
  arc A351 (-33.8878, 0.9525) -> (-32.1122, 0.9525) centre (-33, 0.89) ccw
  arc A352 (-31.8628, 1.22) -> (-32.1122, 0.9525) centre (-31.8628, 0.97) ccw
  line L120 (-31.8628, 1.22) -> (-31.1372, 1.22)
  arc A353 (-30.8878, 0.9525) -> (-31.1372, 1.22) centre (-31.1372, 0.97) ccw
  arc A354 (-30.8878, 0.9525) -> (-29.1122, 0.9525) centre (-30, 0.89) ccw
  arc A355 (-28.8628, 1.22) -> (-29.1122, 0.9525) centre (-28.8628, 0.97) ccw
  line L121 (-28.8628, 1.22) -> (-28.1372, 1.22)
  arc A356 (-27.8878, 0.9525) -> (-28.1372, 1.22) centre (-28.1372, 0.97) ccw
  arc A357 (-27.8878, 0.9525) -> (-26.1122, 0.9525) centre (-27, 0.89) ccw
  arc A358 (-25.8628, 1.22) -> (-26.1122, 0.9525) centre (-25.8628, 0.97) ccw
  line L122 (-25.8628, 1.22) -> (-25.1372, 1.22)
  arc A359 (-24.8878, 0.9525) -> (-25.1372, 1.22) centre (-25.1372, 0.97) ccw
  arc A360 (-24.8878, 0.9525) -> (-23.1122, 0.9525) centre (-24, 0.89) ccw
  arc A361 (-22.8628, 1.22) -> (-23.1122, 0.9525) centre (-22.8628, 0.97) ccw
  line L123 (-22.8628, 1.22) -> (-22.1372, 1.22)
  arc A362 (-21.8878, 0.9525) -> (-22.1372, 1.22) centre (-22.1372, 0.97) ccw
  arc A363 (-21.8878, 0.9525) -> (-20.1122, 0.9525) centre (-21, 0.89) ccw
  arc A364 (-19.8628, 1.22) -> (-20.1122, 0.9525) centre (-19.8628, 0.97) ccw
  line L124 (-19.8628, 1.22) -> (-19.1372, 1.22)
  arc A365 (-18.8878, 0.9525) -> (-19.1372, 1.22) centre (-19.1372, 0.97) ccw
  arc A366 (-18.8878, 0.9525) -> (-17.1122, 0.9525) centre (-18, 0.89) ccw
  arc A367 (-16.8628, 1.22) -> (-17.1122, 0.9525) centre (-16.8628, 0.97) ccw
  line L125 (-16.8628, 1.22) -> (-16.1372, 1.22)
  arc A368 (-15.8878, 0.9525) -> (-16.1372, 1.22) centre (-16.1372, 0.97) ccw
  arc A369 (-15.8878, 0.9525) -> (-14.1122, 0.9525) centre (-15, 0.89) ccw
  arc A370 (-13.8628, 1.22) -> (-14.1122, 0.9525) centre (-13.8628, 0.97) ccw
  line L126 (-13.8628, 1.22) -> (-13.1372, 1.22)
  arc A371 (-12.8878, 0.9525) -> (-13.1372, 1.22) centre (-13.1372, 0.97) ccw
  arc A372 (-12.8878, 0.9525) -> (-11.1122, 0.9525) centre (-12, 0.89) ccw
  arc A373 (-10.8628, 1.22) -> (-11.1122, 0.9525) centre (-10.8628, 0.97) ccw
  line L127 (-10.8628, 1.22) -> (-10.1372, 1.22)
  arc A374 (-9.8878, 0.9525) -> (-10.1372, 1.22) centre (-10.1372, 0.97) ccw
  arc A375 (-9.8878, 0.9525) -> (-8.1122, 0.9525) centre (-9, 0.89) ccw
  arc A376 (-7.8628, 1.22) -> (-8.1122, 0.9525) centre (-7.8628, 0.97) ccw
  line L128 (-7.8628, 1.22) -> (-7.1372, 1.22)
  arc A377 (-6.8878, 0.9525) -> (-7.1372, 1.22) centre (-7.1372, 0.97) ccw
  arc A378 (-6.8878, 0.9525) -> (-5.1122, 0.9525) centre (-6, 0.89) ccw
  arc A379 (-4.8628, 1.22) -> (-5.1122, 0.9525) centre (-4.8628, 0.97) ccw
  line L129 (-4.8628, 1.22) -> (-4.1372, 1.22)
  arc A380 (-3.8878, 0.9525) -> (-4.1372, 1.22) centre (-4.1372, 0.97) ccw
  arc A381 (-3.8878, 0.9525) -> (-2.1122, 0.9525) centre (-3, 0.89) ccw
  arc A382 (-1.8628, 1.22) -> (-2.1122, 0.9525) centre (-1.8628, 0.97) ccw
  line L130 (-1.8628, 1.22) -> (-1.1372, 1.22)
  arc A383 (-0.8878, 0.9525) -> (-1.1372, 1.22) centre (-1.1372, 0.97) ccw
  arc A384 (-0.8878, 0.9525) -> (0, 0) centre (0, 0.89) ccw
  line L131 (-768, 0) -> (-768, 2.4)
  line L132 (-768, 2.4) -> (-384, 2.4)
  arc A385 (-384.8878, 0.9525) -> (-384, 0) centre (-384, 0.89) ccw
  arc A386 (-384.8878, 0.9525) -> (-385.1372, 1.22) centre (-385.1372, 0.97) ccw
  line L133 (-385.1372, 1.22) -> (-385.8628, 1.22)
  arc A387 (-385.8628, 1.22) -> (-386.1122, 0.9525) centre (-385.8628, 0.97) ccw
  arc A388 (-387.8878, 0.9525) -> (-386.1122, 0.9525) centre (-387, 0.89) ccw
  arc A389 (-387.8878, 0.9525) -> (-388.1372, 1.22) centre (-388.1372, 0.97) ccw
  line L134 (-388.1372, 1.22) -> (-388.8628, 1.22)
  arc A390 (-388.8628, 1.22) -> (-389.1122, 0.9525) centre (-388.8628, 0.97) ccw
  arc A391 (-390.8878, 0.9525) -> (-389.1122, 0.9525) centre (-390, 0.89) ccw
  arc A392 (-390.8878, 0.9525) -> (-391.1372, 1.22) centre (-391.1372, 0.97) ccw
  line L135 (-391.1372, 1.22) -> (-391.8628, 1.22)
  arc A393 (-391.8628, 1.22) -> (-392.1122, 0.9525) centre (-391.8628, 0.97) ccw
  arc A394 (-393.8878, 0.9525) -> (-392.1122, 0.9525) centre (-393, 0.89) ccw
  arc A395 (-393.8878, 0.9525) -> (-394.1372, 1.22) centre (-394.1372, 0.97) ccw
  line L136 (-394.1372, 1.22) -> (-394.8628, 1.22)
  arc A396 (-394.8628, 1.22) -> (-395.1122, 0.9525) centre (-394.8628, 0.97) ccw
  arc A397 (-396.8878, 0.9525) -> (-395.1122, 0.9525) centre (-396, 0.89) ccw
  arc A398 (-396.8878, 0.9525) -> (-397.1372, 1.22) centre (-397.1372, 0.97) ccw
  line L137 (-397.1372, 1.22) -> (-397.8628, 1.22)
  arc A399 (-397.8628, 1.22) -> (-398.1122, 0.9525) centre (-397.8628, 0.97) ccw
  arc A400 (-399.8878, 0.9525) -> (-398.1122, 0.9525) centre (-399, 0.89) ccw
  arc A401 (-399.8878, 0.9525) -> (-400.1372, 1.22) centre (-400.1372, 0.97) ccw
  line L138 (-400.1372, 1.22) -> (-400.8628, 1.22)
  arc A402 (-400.8628, 1.22) -> (-401.1122, 0.9525) centre (-400.8628, 0.97) ccw
  arc A403 (-402.8878, 0.9525) -> (-401.1122, 0.9525) centre (-402, 0.89) ccw
  arc A404 (-402.8878, 0.9525) -> (-403.1372, 1.22) centre (-403.1372, 0.97) ccw
  line L139 (-403.1372, 1.22) -> (-403.8628, 1.22)
  arc A405 (-403.8628, 1.22) -> (-404.1122, 0.9525) centre (-403.8628, 0.97) ccw
  arc A406 (-405.8878, 0.9525) -> (-404.1122, 0.9525) centre (-405, 0.89) ccw
  arc A407 (-405.8878, 0.9525) -> (-406.1372, 1.22) centre (-406.1372, 0.97) ccw
  line L140 (-406.1372, 1.22) -> (-406.8628, 1.22)
  arc A408 (-406.8628, 1.22) -> (-407.1122, 0.9525) centre (-406.8628, 0.97) ccw
  arc A409 (-408.8878, 0.9525) -> (-407.1122, 0.9525) centre (-408, 0.89) ccw
  arc A410 (-408.8878, 0.9525) -> (-409.1372, 1.22) centre (-409.1372, 0.97) ccw
  line L141 (-409.1372, 1.22) -> (-409.8628, 1.22)
  arc A411 (-409.8628, 1.22) -> (-410.1122, 0.9525) centre (-409.8628, 0.97) ccw
  arc A412 (-411.8878, 0.9525) -> (-410.1122, 0.9525) centre (-411, 0.89) ccw
  arc A413 (-411.8878, 0.9525) -> (-412.1372, 1.22) centre (-412.1372, 0.97) ccw
  line L142 (-412.1372, 1.22) -> (-412.8628, 1.22)
  arc A414 (-412.8628, 1.22) -> (-413.1122, 0.9525) centre (-412.8628, 0.97) ccw
  arc A415 (-414.8878, 0.9525) -> (-413.1122, 0.9525) centre (-414, 0.89) ccw
  arc A416 (-414.8878, 0.9525) -> (-415.1372, 1.22) centre (-415.1372, 0.97) ccw
  line L143 (-415.1372, 1.22) -> (-415.8628, 1.22)
  arc A417 (-415.8628, 1.22) -> (-416.1122, 0.9525) centre (-415.8628, 0.97) ccw
  arc A418 (-417.8878, 0.9525) -> (-416.1122, 0.9525) centre (-417, 0.89) ccw
  arc A419 (-417.8878, 0.9525) -> (-418.1372, 1.22) centre (-418.1372, 0.97) ccw
  line L144 (-418.1372, 1.22) -> (-418.8628, 1.22)
  arc A420 (-418.8628, 1.22) -> (-419.1122, 0.9525) centre (-418.8628, 0.97) ccw
  arc A421 (-420.8878, 0.9525) -> (-419.1122, 0.9525) centre (-420, 0.89) ccw
  arc A422 (-420.8878, 0.9525) -> (-421.1372, 1.22) centre (-421.1372, 0.97) ccw
  line L145 (-421.1372, 1.22) -> (-421.8628, 1.22)
  arc A423 (-421.8628, 1.22) -> (-422.1122, 0.9525) centre (-421.8628, 0.97) ccw
  arc A424 (-423.8878, 0.9525) -> (-422.1122, 0.9525) centre (-423, 0.89) ccw
  arc A425 (-423.8878, 0.9525) -> (-424.1372, 1.22) centre (-424.1372, 0.97) ccw
  line L146 (-424.1372, 1.22) -> (-424.8628, 1.22)
  arc A426 (-424.8628, 1.22) -> (-425.1122, 0.9525) centre (-424.8628, 0.97) ccw
  arc A427 (-426.8878, 0.9525) -> (-425.1122, 0.9525) centre (-426, 0.89) ccw
  arc A428 (-426.8878, 0.9525) -> (-427.1372, 1.22) centre (-427.1372, 0.97) ccw
  line L147 (-427.1372, 1.22) -> (-427.8628, 1.22)
  arc A429 (-427.8628, 1.22) -> (-428.1122, 0.9525) centre (-427.8628, 0.97) ccw
  arc A430 (-429.8878, 0.9525) -> (-428.1122, 0.9525) centre (-429, 0.89) ccw
  arc A431 (-429.8878, 0.9525) -> (-430.1372, 1.22) centre (-430.1372, 0.97) ccw
  line L148 (-430.1372, 1.22) -> (-430.8628, 1.22)
  arc A432 (-430.8628, 1.22) -> (-431.1122, 0.9525) centre (-430.8628, 0.97) ccw
  arc A433 (-432.8878, 0.9525) -> (-431.1122, 0.9525) centre (-432, 0.89) ccw
  arc A434 (-432.8878, 0.9525) -> (-433.1372, 1.22) centre (-433.1372, 0.97) ccw
  line L149 (-433.1372, 1.22) -> (-433.8628, 1.22)
  arc A435 (-433.8628, 1.22) -> (-434.1122, 0.9525) centre (-433.8628, 0.97) ccw
  arc A436 (-435.8878, 0.9525) -> (-434.1122, 0.9525) centre (-435, 0.89) ccw
  arc A437 (-435.8878, 0.9525) -> (-436.1372, 1.22) centre (-436.1372, 0.97) ccw
  line L150 (-436.1372, 1.22) -> (-436.8628, 1.22)
  arc A438 (-436.8628, 1.22) -> (-437.1122, 0.9525) centre (-436.8628, 0.97) ccw
  arc A439 (-438.8878, 0.9525) -> (-437.1122, 0.9525) centre (-438, 0.89) ccw
  arc A440 (-438.8878, 0.9525) -> (-439.1372, 1.22) centre (-439.1372, 0.97) ccw
  line L151 (-439.1372, 1.22) -> (-439.8628, 1.22)
  arc A441 (-439.8628, 1.22) -> (-440.1122, 0.9525) centre (-439.8628, 0.97) ccw
  arc A442 (-441.8878, 0.9525) -> (-440.1122, 0.9525) centre (-441, 0.89) ccw
  arc A443 (-441.8878, 0.9525) -> (-442.1372, 1.22) centre (-442.1372, 0.97) ccw
  line L152 (-442.1372, 1.22) -> (-442.8628, 1.22)
  arc A444 (-442.8628, 1.22) -> (-443.1122, 0.9525) centre (-442.8628, 0.97) ccw
  arc A445 (-444.8878, 0.9525) -> (-443.1122, 0.9525) centre (-444, 0.89) ccw
  arc A446 (-444.8878, 0.9525) -> (-445.1372, 1.22) centre (-445.1372, 0.97) ccw
  line L153 (-445.1372, 1.22) -> (-445.8628, 1.22)
  arc A447 (-445.8628, 1.22) -> (-446.1122, 0.9525) centre (-445.8628, 0.97) ccw
  arc A448 (-447.8878, 0.9525) -> (-446.1122, 0.9525) centre (-447, 0.89) ccw
  arc A449 (-447.8878, 0.9525) -> (-448.1372, 1.22) centre (-448.1372, 0.97) ccw
  line L154 (-448.1372, 1.22) -> (-448.8628, 1.22)
  arc A450 (-448.8628, 1.22) -> (-449.1122, 0.9525) centre (-448.8628, 0.97) ccw
  arc A451 (-450.8878, 0.9525) -> (-449.1122, 0.9525) centre (-450, 0.89) ccw
  arc A452 (-450.8878, 0.9525) -> (-451.1372, 1.22) centre (-451.1372, 0.97) ccw
  line L155 (-451.1372, 1.22) -> (-451.8628, 1.22)
  arc A453 (-451.8628, 1.22) -> (-452.1122, 0.9525) centre (-451.8628, 0.97) ccw
  arc A454 (-453.8878, 0.9525) -> (-452.1122, 0.9525) centre (-453, 0.89) ccw
  arc A455 (-453.8878, 0.9525) -> (-454.1372, 1.22) centre (-454.1372, 0.97) ccw
  line L156 (-454.1372, 1.22) -> (-454.8628, 1.22)
  arc A456 (-454.8628, 1.22) -> (-455.1122, 0.9525) centre (-454.8628, 0.97) ccw
  arc A457 (-456.8878, 0.9525) -> (-455.1122, 0.9525) centre (-456, 0.89) ccw
  arc A458 (-456.8878, 0.9525) -> (-457.1372, 1.22) centre (-457.1372, 0.97) ccw
  line L157 (-457.1372, 1.22) -> (-457.8628, 1.22)
  arc A459 (-457.8628, 1.22) -> (-458.1122, 0.9525) centre (-457.8628, 0.97) ccw
  arc A460 (-459.8878, 0.9525) -> (-458.1122, 0.9525) centre (-459, 0.89) ccw
  arc A461 (-459.8878, 0.9525) -> (-460.1372, 1.22) centre (-460.1372, 0.97) ccw
  line L158 (-460.1372, 1.22) -> (-460.8628, 1.22)
  arc A462 (-460.8628, 1.22) -> (-461.1122, 0.9525) centre (-460.8628, 0.97) ccw
  arc A463 (-462.8878, 0.9525) -> (-461.1122, 0.9525) centre (-462, 0.89) ccw
  arc A464 (-462.8878, 0.9525) -> (-463.1372, 1.22) centre (-463.1372, 0.97) ccw
  line L159 (-463.1372, 1.22) -> (-463.8628, 1.22)
  arc A465 (-463.8628, 1.22) -> (-464.1122, 0.9525) centre (-463.8628, 0.97) ccw
  arc A466 (-465.8878, 0.9525) -> (-464.1122, 0.9525) centre (-465, 0.89) ccw
  arc A467 (-465.8878, 0.9525) -> (-466.1372, 1.22) centre (-466.1372, 0.97) ccw
  line L160 (-466.1372, 1.22) -> (-466.8628, 1.22)
  arc A468 (-466.8628, 1.22) -> (-467.1122, 0.9525) centre (-466.8628, 0.97) ccw
  arc A469 (-468.8878, 0.9525) -> (-467.1122, 0.9525) centre (-468, 0.89) ccw
  arc A470 (-468.8878, 0.9525) -> (-469.1372, 1.22) centre (-469.1372, 0.97) ccw
  line L161 (-469.1372, 1.22) -> (-469.8628, 1.22)
  arc A471 (-469.8628, 1.22) -> (-470.1122, 0.9525) centre (-469.8628, 0.97) ccw
  arc A472 (-471.8878, 0.9525) -> (-470.1122, 0.9525) centre (-471, 0.89) ccw
  arc A473 (-471.8878, 0.9525) -> (-472.1372, 1.22) centre (-472.1372, 0.97) ccw
  line L162 (-472.1372, 1.22) -> (-472.8628, 1.22)
  arc A474 (-472.8628, 1.22) -> (-473.1122, 0.9525) centre (-472.8628, 0.97) ccw
  arc A475 (-474.8878, 0.9525) -> (-473.1122, 0.9525) centre (-474, 0.89) ccw
  arc A476 (-474.8878, 0.9525) -> (-475.1372, 1.22) centre (-475.1372, 0.97) ccw
  line L163 (-475.1372, 1.22) -> (-475.8628, 1.22)
  arc A477 (-475.8628, 1.22) -> (-476.1122, 0.9525) centre (-475.8628, 0.97) ccw
  arc A478 (-477.8878, 0.9525) -> (-476.1122, 0.9525) centre (-477, 0.89) ccw
  arc A479 (-477.8878, 0.9525) -> (-478.1372, 1.22) centre (-478.1372, 0.97) ccw
  line L164 (-478.1372, 1.22) -> (-478.8628, 1.22)
  arc A480 (-478.8628, 1.22) -> (-479.1122, 0.9525) centre (-478.8628, 0.97) ccw
  arc A481 (-480.8878, 0.9525) -> (-479.1122, 0.9525) centre (-480, 0.89) ccw
  arc A482 (-480.8878, 0.9525) -> (-481.1372, 1.22) centre (-481.1372, 0.97) ccw
  line L165 (-481.1372, 1.22) -> (-481.8628, 1.22)
  arc A483 (-481.8628, 1.22) -> (-482.1122, 0.9525) centre (-481.8628, 0.97) ccw
  arc A484 (-483.8878, 0.9525) -> (-482.1122, 0.9525) centre (-483, 0.89) ccw
  arc A485 (-483.8878, 0.9525) -> (-484.1372, 1.22) centre (-484.1372, 0.97) ccw
  line L166 (-484.1372, 1.22) -> (-484.8628, 1.22)
  arc A486 (-484.8628, 1.22) -> (-485.1122, 0.9525) centre (-484.8628, 0.97) ccw
  arc A487 (-486.8878, 0.9525) -> (-485.1122, 0.9525) centre (-486, 0.89) ccw
  arc A488 (-486.8878, 0.9525) -> (-487.1372, 1.22) centre (-487.1372, 0.97) ccw
  line L167 (-487.1372, 1.22) -> (-487.8628, 1.22)
  arc A489 (-487.8628, 1.22) -> (-488.1122, 0.9525) centre (-487.8628, 0.97) ccw
  arc A490 (-489.8878, 0.9525) -> (-488.1122, 0.9525) centre (-489, 0.89) ccw
  arc A491 (-489.8878, 0.9525) -> (-490.1372, 1.22) centre (-490.1372, 0.97) ccw
  line L168 (-490.1372, 1.22) -> (-490.8628, 1.22)
  arc A492 (-490.8628, 1.22) -> (-491.1122, 0.9525) centre (-490.8628, 0.97) ccw
  arc A493 (-492.8878, 0.9525) -> (-491.1122, 0.9525) centre (-492, 0.89) ccw
  arc A494 (-492.8878, 0.9525) -> (-493.1372, 1.22) centre (-493.1372, 0.97) ccw
  line L169 (-493.1372, 1.22) -> (-493.8628, 1.22)
  arc A495 (-493.8628, 1.22) -> (-494.1122, 0.9525) centre (-493.8628, 0.97) ccw
  arc A496 (-495.8878, 0.9525) -> (-494.1122, 0.9525) centre (-495, 0.89) ccw
  arc A497 (-495.8878, 0.9525) -> (-496.1372, 1.22) centre (-496.1372, 0.97) ccw
  line L170 (-496.1372, 1.22) -> (-496.8628, 1.22)
  arc A498 (-496.8628, 1.22) -> (-497.1122, 0.9525) centre (-496.8628, 0.97) ccw
  arc A499 (-498.8878, 0.9525) -> (-497.1122, 0.9525) centre (-498, 0.89) ccw
  arc A500 (-498.8878, 0.9525) -> (-499.1372, 1.22) centre (-499.1372, 0.97) ccw
  line L171 (-499.1372, 1.22) -> (-499.8628, 1.22)
  arc A501 (-499.8628, 1.22) -> (-500.1122, 0.9525) centre (-499.8628, 0.97) ccw
  arc A502 (-501.8878, 0.9525) -> (-500.1122, 0.9525) centre (-501, 0.89) ccw
  arc A503 (-501.8878, 0.9525) -> (-502.1372, 1.22) centre (-502.1372, 0.97) ccw
  line L172 (-502.1372, 1.22) -> (-502.8628, 1.22)
  arc A504 (-502.8628, 1.22) -> (-503.1122, 0.9525) centre (-502.8628, 0.97) ccw
  arc A505 (-504.8878, 0.9525) -> (-503.1122, 0.9525) centre (-504, 0.89) ccw
  arc A506 (-504.8878, 0.9525) -> (-505.1372, 1.22) centre (-505.1372, 0.97) ccw
  line L173 (-505.1372, 1.22) -> (-505.8628, 1.22)
  arc A507 (-505.8628, 1.22) -> (-506.1122, 0.9525) centre (-505.8628, 0.97) ccw
  arc A508 (-507.8878, 0.9525) -> (-506.1122, 0.9525) centre (-507, 0.89) ccw
  arc A509 (-507.8878, 0.9525) -> (-508.1372, 1.22) centre (-508.1372, 0.97) ccw
  line L174 (-508.1372, 1.22) -> (-508.8628, 1.22)
  arc A510 (-508.8628, 1.22) -> (-509.1122, 0.9525) centre (-508.8628, 0.97) ccw
  arc A511 (-510.8878, 0.9525) -> (-509.1122, 0.9525) centre (-510, 0.89) ccw
  arc A512 (-510.8878, 0.9525) -> (-511.1372, 1.22) centre (-511.1372, 0.97) ccw
  line L175 (-511.1372, 1.22) -> (-511.8628, 1.22)
  arc A513 (-511.8628, 1.22) -> (-512.1122, 0.9525) centre (-511.8628, 0.97) ccw
  arc A514 (-513.8878, 0.9525) -> (-512.1122, 0.9525) centre (-513, 0.89) ccw
  arc A515 (-513.8878, 0.9525) -> (-514.1372, 1.22) centre (-514.1372, 0.97) ccw
  line L176 (-514.1372, 1.22) -> (-514.8628, 1.22)
  arc A516 (-514.8628, 1.22) -> (-515.1122, 0.9525) centre (-514.8628, 0.97) ccw
  arc A517 (-516.8878, 0.9525) -> (-515.1122, 0.9525) centre (-516, 0.89) ccw
  arc A518 (-516.8878, 0.9525) -> (-517.1372, 1.22) centre (-517.1372, 0.97) ccw